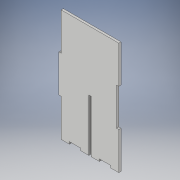
# Autodesk Inventor part: Pared Garita2
Saved by Autodesk Inventor 2019 (Build 230136000, 136)
## iProperties
Created: 2020-03-09
Part Number: Pared Garita2
Material: Genérico
Document SubType Name: Modeling
Designer: Diego Guillén
Density: 1 g/cm^3
Appearance: Valor por defecto
Author: Diego Guillén
Autodesk Inventor part; units mm, degrees
ref_plane "YZ Plane" through (0, 0, 0) normal (1, 0, 0) x (0, 1, 0)
ref_plane "XZ Plane" through (0, 0, 0) normal (0, 1, 0) x (-1, 0, 0)
ref_plane "XY Plane" through (0, 0, 0) normal (0, 0, 1) x (1, 0, 0)
sketch "Boceto1" plane through (0, 0, 0) normal (0, 0, 1) x (1, 0, 0)
  line L0 (0, 0) -> (80, 0)
  line L1 (80, 0) -> (80, 150)
  line L2 (80, 150) -> (0, 150)
  line L3 (0, 150) -> (0, 0)
  dimension "d0" = 80
  dimension "d1" = 150
  constraints: 8 end point, 2 parallel, 1 horizontal, 1 perpendicular
  measures "d0" distance of L1.end L2.end
  measures "d1" distance of L0.end L1.end
extrude "Extrusión1" add sketch "Boceto1" along normal blind 3
sketch "Boceto2" plane through (0, 0, 3) normal (0, 0, 1) x (1, 0, 0)
  line L0 (0, 0) -> (80, 0) construction
  line L1 (80, 0) -> (80, 150) construction
  line L2 (80, 150) -> (0, 150) construction
  line L3 (0, 150) -> (0, 0) construction
  line L4 (3, 0) -> (0, 0)
  line L5 (0, 0) -> (0, 50)
  line L6 (0, 50) -> (3, 50)
  line L7 (3, 50) -> (3, 0)
  line L8 (0, 150) -> (3, 150)
  line L9 (3, 150) -> (3, 100)
  line L10 (3, 100) -> (0, 100)
  line L11 (0, 100) -> (0, 150)
  line L12 (77, 100) -> (80, 100)
  line L13 (80, 100) -> (80, 50)
  line L14 (80, 50) -> (77, 50)
  line L15 (77, 50) -> (77, 100)
  line L16 (80, 0) -> (80, 150) construction
  point P0 (80, 75)
  point P1 (80, 75)
  dimension "d4" = 3
  dimension "d5" = 50
  dimension "d6" = 3
  dimension "d7" = 50
  dimension "d8" = 50
  dimension "d9" = 3
  constraints: 24 end point, 6 parallel, 3 horizontal, 3 perpendicular, 2 coincident, 2 midpoint, 1 collinear
  measures "d4" distance of L5.end L6.end
  measures "d5" distance of L6.end L4.start
  measures "d6" distance of L9.end L10.end
  measures "d7" distance of L8.end L9.end
  measures "d8" distance of L14.end L12.start
  measures "d9" distance of L13.end L14.end
extrude "Extrusión2" cut sketch "Boceto2" against normal blind 3
sketch "Boceto3" plane through (0, 0, 3) normal (0, 0, 1) x (1, 0, 0)
  line L0 (3, 50) -> (3, 0) construction
  line L1 (3, 0) -> (80, 0) construction
  line L2 (80, 0) -> (80, 50) construction
  line L3 (80, 50) -> (77, 50) construction
  line L4 (77, 50) -> (77, 100) construction
  line L5 (77, 100) -> (80, 100) construction
  line L6 (80, 100) -> (80, 150) construction
  line L7 (80, 150) -> (3, 150) construction
  line L8 (3, 150) -> (3, 100) construction
  line L9 (3, 100) -> (0, 100) construction
  line L10 (0, 100) -> (0, 50) construction
  line L11 (0, 50) -> (3, 50) construction
  line L12 (40, 70) -> (43, 70)
  line L13 (43, 70) -> (43, 0)
  line L14 (43, 0) -> (40, 0)
  line L15 (40, 0) -> (40, 70)
  line L16 (3, 0) -> (80, 0) construction
  point P0 (0, 0)
  point P1 (41.5, 0)
  point P2 (41.5, 0)
  dimension "d12" = 3
  dimension "d13" = 70
  constraints: 8 end point, 2 midpoint, 2 parallel, 1 coincident, 1 collinear, 1 horizontal, 1 perpendicular
  measures "d12" distance of L13.end L14.end
  measures "d13" distance of L14.end L12.start
extrude "Extrusión3" cut sketch "Boceto3" against normal blind 10
sketch "Boceto4" plane through (0, 0, 3) normal (0, 0, 1) x (1, 0, 0)
  line L0 (43, 70) -> (43, 0) construction
  line L1 (43, 0) -> (80, 0) construction
  line L2 (80, 0) -> (80, 50) construction
  line L3 (80, 50) -> (77, 50) construction
  line L4 (77, 50) -> (77, 100) construction
  line L5 (77, 100) -> (80, 100) construction
  line L6 (80, 100) -> (80, 150) construction
  line L7 (80, 150) -> (3, 150) construction
  line L8 (3, 150) -> (3, 100) construction
  line L9 (3, 100) -> (0, 100) construction
  line L10 (0, 100) -> (0, 50) construction
  line L11 (0, 50) -> (3, 50) construction
  line L12 (3, 50) -> (3, 0) construction
  line L13 (3, 0) -> (40, 0) construction
  line L14 (40, 0) -> (40, 70) construction
  line L15 (40, 70) -> (43, 70) construction
  line L16 (14, 3) -> (29, 3)
  line L17 (29, 3) -> (29, 0)
  line L18 (29, 0) -> (14, 0)
  line L19 (14, 0) -> (14, 3)
  line L20 (69, 3) -> (54, 3)
  line L21 (54, 3) -> (54, 0)
  line L22 (54, 0) -> (69, 0)
  line L23 (69, 0) -> (69, 3)
  line L24 (3, 0) -> (40, 0) construction
  point P0 (0, 0)
  point P1 (61.5, 0)
  point P2 (61.5, 0)
  point P3 (21.5, 0)
  point P4 (21.5, 0)
  dimension "d16" = 3
  dimension "d17" = 3
  dimension "d18" = 15
  dimension "d19" = 15
  constraints: 16 end point, 4 midpoint, 4 parallel, 2 coincident, 2 horizontal, 2 perpendicular, 1 collinear, 1 point on line
  measures "d16" distance of L18.end L16.start
  measures "d17" distance of L20.end L21.end
  measures "d18" distance of L16.start L16.end
  measures "d19" distance of L20.start L20.end
extrude "Extrusión4" cut sketch "Boceto4" against normal blind 10
equation "\"d6\" = d4"
equation "\"d7\" = d5"
equation "\"d8\" = d7"
equation "\"d9\" = d4"
equation "\"d19\" = d18"
